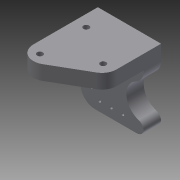
# Autodesk Inventor part: joint3+ax12imprint_v4
Saved by Autodesk Inventor 2014 (Build 180170000, 170)
## iProperties
Created: 2014-01-23
Part Number: joint3+ax12imprint_v4
Material: Générique
Document SubType Name: Modeling
Designer: helly
Density: 1 g/cm^3
Appearance: Par défaut
Author: helly
Autodesk Inventor part; units mm, degrees
note: some values were not read from the file. Chosen so that the rebuilt part matches the saved one: edges of "Congé5".
ref_plane "YZ Plane" through (0, 0, 0) normal (1, 0, 0) x (0, 1, 0)
ref_plane "XZ Plane" through (0, 0, 0) normal (0, 1, 0) x (-1, 0, 0)
ref_plane "XY Plane" through (0, 0, 0) normal (0, 0, 1) x (1, 0, 0)
sketch "Esquisse1" plane through (0, 0, 0) normal (0, 0, 1) x (1, 0, 0)
  line L0 (0, 0) -> (0, 32) construction
  line L1 (0, 32) -> (27.7128, 16) construction
  line L2 (27.7128, 16) -> (0, 0) construction
  circle A0 centre (0, 0) radius 2
  circle A1 centre (0, 32) radius 2
  circle A2 centre (27.7128, 16) radius 2
  line L3 (0, 32) -> (0, 48) construction
  line L4 (35.7128, 48) -> (35.7128, 11.3812)
  line L5 (2.1436, -8) -> (-8, -8)
  line L6 (-8, -8) -> (-8, 48)
  line L7 (-8, 48) -> (35.7128, 48)
  line L8 (27.7128, 16) -> (35.7128, 16) construction
  line L9 (0, 0) -> (0, -8) construction
  line L10 (0, 32) -> (-8, 32) construction
  line L11 (27.7128, 16) -> (31.7128, 9.0718) construction
  line L12 (35.7128, 11.3812) -> (2.1436, -8)
  dimension "d0" = 32
  dimension "d1" = 32
  dimension "d2" = 32
  dimension "d3" = 4
  dimension "d4" = 16
  dimension "d5" = 8
  dimension "d6" = 8
  dimension "d7" = 8
  dimension "d27" = 8
  constraints: 26 end point, 5 point on line, 4 parallel, 4 perpendicular, 3 centre point, 3 coincident, 2 collinear, 2 equal radius, 1 vertical
  measures "d0" distance of L0.start L0.end
  measures "d1" distance of L0.end L1.end
  measures "d2" distance of L0.start L1.end
  measures "d3" diameter of A0
  measures "d4" distance of L3.start L3.end
  measures "d5" distance of L8.start L8.end
  measures "d6" distance of L9.start L9.end
  measures "d7" distance of L3.start L10.end
  measures "d27" distance of L8.start L11.end
extrude "Extrusion1" add sketch "Esquisse1" along normal blind 10
sketch "Esquisse2" plane through (0, 0, 0) normal (0, 0, -1) x (-1, 0, 0)
  circle A0 centre (-27.7128, 16) radius 2 projected
  circle A1 centre (0, 32) radius 2 projected
  circle A2 centre (0, 0) radius 2 projected
  line L0 (-35.7128, 48) -> (-35.7128, -8) projected
  line L1 (8, -8) -> (8, 48) projected
  line L2 (8, 48) -> (-35.7128, 48) projected
  line L3 (0, 27.9585) -> (-3.5, 29.9793)
  line L4 (-3.5, 29.9793) -> (-3.5, 34.0207)
  line L5 (-3.5, 34.0207) -> (0, 36.0415)
  line L6 (0, 36.0415) -> (3.5, 34.0207)
  line L7 (3.5, 34.0207) -> (3.5, 29.9793)
  line L8 (3.5, 29.9793) -> (0, 27.9585)
  line L9 (-3.5, 2.0207) -> (0, 4.0415)
  line L10 (0, 4.0415) -> (3.5, 2.0207)
  line L11 (3.5, 2.0207) -> (3.5, -2.0207)
  line L12 (3.5, -2.0207) -> (0, -4.0415)
  line L13 (0, -4.0415) -> (-3.5, -2.0207)
  line L14 (-3.5, -2.0207) -> (-3.5, 2.0207)
  line L15 (-3.5, 29.9793) -> (3.5, 29.9793) construction
  line L16 (-24.2128, 13.9793) -> (-27.7128, 11.9585)
  line L17 (-27.7128, 11.9585) -> (-31.2128, 13.9793)
  line L18 (-31.2128, 13.9793) -> (-31.2128, 18.0207)
  line L19 (-31.2128, 18.0207) -> (-27.7128, 20.0415)
  line L20 (-27.7128, 20.0415) -> (-24.2128, 18.0207)
  line L21 (-24.2128, 18.0207) -> (-24.2128, 13.9793)
  point P0 (-2.1436, -8)
  dimension "d10" = 7
  constraints: 38 end point, 4 coincident, 3 parallel, 2 equal length, 39 other
  measures "d10" distance of L3.end L7.end
extrude "Extrusion2" cut sketch "Esquisse2" against normal blind 3
sketch "Esquisse5" plane through (0, 0, 0) normal (0, 0, -1) x (-1, 0, 0)
  line L0 (-35.7128, 48) -> (-35.7128, 11.3812) projected
  line L1 (8, -8) -> (8, 48) projected
  line L2 (8, 48) -> (-35.7128, 48) projected
  line L3 (-35.7128, 48) -> (8, 48)
  line L4 (8, 48) -> (8, 36)
  line L5 (8, 36) -> (-35.7128, 36)
  line L6 (-35.7128, 36) -> (-35.7128, 48)
  point P0 (0, 0)
  dimension "d28" = 12
  constraints: 8 end point, 2 collinear, 2 point on line, 1 perpendicular
  measures "d28" distance of L1.end L4.end
extrude "Extrusion5" add sketch "Esquisse5" along normal blind 40
sketch "Esquisse6" plane through (0.0718, 36, 0) normal (0, -1, 0) x (1, 0, 0)
  line L0 (-8.0718, 0) -> (-8.0718, -40) projected
  line L1 (35.641, 0) -> (35.641, -40) projected
  line L2 (35.641, -20) -> (-8.0718, -20) construction
  circle A0 centre (35.641, -20) radius 12
  line L3 (35.641, -20) -> (35.641, -6.5) construction
  line L4 (35.641, -6.5) -> (29.141, -6.5) construction
  line L5 (29.141, -6.5) -> (21.141, -6.5) construction
  line L6 (21.141, -6.5) -> (13.141, -6.5) construction
  line L7 (13.141, -6.5) -> (5.141, -6.5) construction
  line L8 (35.641, -20) -> (-0.359, -20) construction
  line L9 (-0.359, -20) -> (-0.359, -12) construction
  circle A1 centre (-0.359, -12) radius 1
  circle A2 centre (5.141, -6.5) radius 1
  circle A3 centre (13.141, -6.5) radius 1
  circle A4 centre (21.141, -6.5) radius 1
  circle A5 centre (-0.359, -28) radius 1
  circle A6 centre (5.141, -33.5) radius 1
  circle A7 centre (13.141, -33.5) radius 1
  circle A8 centre (21.141, -33.5) radius 1
  point P0 (-0.0718, 0)
  dimension "d31" = 24
  dimension "d32" = 13.5
  dimension "d33" = 6.5
  dimension "d34" = 8
  dimension "d35" = 8
  dimension "d36" = 8
  dimension "d37" = 36
  dimension "d38" = 8
  dimension "d39" = 2
  constraints: 16 end point, 9 centre point, 5 coincident, 5 perpendicular, 4 symmetric about line, 3 equal radius, 2 midpoint, 2 point on line, 4 other
  measures "d31" diameter of A0
  measures "d32" distance of L3.start L3.end
  measures "d33" distance of L3.end L4.end
  measures "d34" distance of L4.end L5.end
  measures "d35" distance of L5.end L6.end
  measures "d36" distance of L6.end L7.end
  measures "d37" distance of L3.start L8.end
  measures "d38" distance of L8.end L9.end
  measures "d39" diameter of A1
extrude "Extrusion6" cut sketch "Esquisse6" against normal through all
fillet "Congé1" radius 10 1 edges at (-8, -8, 5)
fillet "Congé2" radius 10 1 edges at (35.7128, 11.3812, 5)
fillet "Congé3" radius 10 1 edges at (2.1436, -8, 5)
fillet "Congé4" radius 10 1 edges at (-8, 42, -40)
fillet "Congé5" radius 10 1 edges at (35.7128, 42, -8)
fillet "Congé6" radius 5 1 edges at (35.7128, 42, -32)
fillet "Congé7" radius 5 1 edges at (35.7128, 42, -40)
